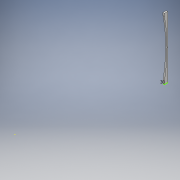
# Autodesk Inventor part: Group Bridge
Saved by Autodesk Inventor 2018 (Build 220112000, 112)
## iProperties
Created: 2018-05-02
Part Number: Group Bridge
Material: Generic
Document SubType Name: Modeling
Designer: Owner
Density: 1 g/cm^3
Appearance: Default
Author: Owner
Autodesk Inventor part; units mm, degrees
ref_plane "YZ Plane" through (0, 0, 0) normal (1, 0, 0) x (0, 1, 0)
ref_plane "XZ Plane" through (0, 0, 0) normal (0, 1, 0) x (-1, 0, 0)
ref_plane "XY Plane" through (0, 0, 0) normal (0, 0, 1) x (1, 0, 0)
sketch "Sketch1" plane through (0, 0, 0) normal (0, 0, 1) x (1, 0, 0)
  line L0 (-7.8997, 15.5643) -> (8.1818, 15.5643)
  line L1 (8.1818, 15.5643) -> (8.1818, -14.4357)
  line L2 (8.1818, -14.4357) -> (-7.8997, -14.4357)
  line L3 (-7.8997, -14.4357) -> (-7.8997, 15.5643)
  line L4 (8.1818, 15.5643) -> (-7.8997, 15.5643)
  line L5 (-7.8997, 15.5643) -> (-7.8997, 23.2199)
  line L6 (-7.8997, 23.2199) -> (8.1818, 23.2199)
  line L7 (8.1818, 23.2199) -> (8.1818, 15.5643)
  point P0 (0, 0)
  dimension "d6" = 30
  constraints: 16 end point, 4 parallel, 2 horizontal, 2 perpendicular
  measures "d6" distance of L2.end L0.start
extrude "Extrusion1" add sketch "Sketch1" along normal blind 700 contours L0 L1 L2 L3
sketch "Sketch2" plane through (8.1818, -14.4357, 0) normal (1, 0, 0) x (0, 0, -1)
  line L0 (0, 0) -> (-700, 0) projected
  arc A0 (-30, 0) -> (-670, 0) centre (-350, -1691.6667) ccw
  line L1 (-30, 0) -> (-670, 0)
  line L2 (0, 30) -> (-700, 30) projected
  point P0 (0, 14.4357)
  dimension "d4" = 30
  dimension "d5" = 30
  constraints: 2 end point, 2 point on circle, 1 centre point, 1 collinear, 1 point on line, 1 tangent
  measures "d4" distance of L0.start L1.start
  measures "d5" distance of L0.end L1.end
extrude "Extrusion2" cut sketch "Sketch2" against normal blind 90000
sketch "Sketch3" plane through (0, 0, 0) normal (0, 0, -1) x (-1, 0, 0)
  point P0 (0, 0)
extrude "Extrusion3" add sketch "Sketch1" along normal up to surface (700 mm away) contours L5 L6 L7 L0
equation "\"d5\" = d4"
body "Solid1"
